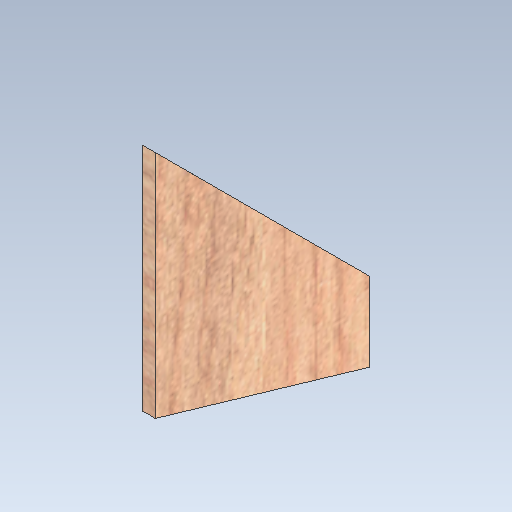
# Autodesk Inventor part: Aletas
Saved by Autodesk Inventor 2020 (Build 240168000, 168)
## iProperties
Created: 2021-10-16
Part Number: Aletas
Material: Birch
Document SubType Name: Modeling
Designer: Carlos
Density: 0.512 g/cm^3
Appearance: Birch - Natural Medium Gloss
Mass: 12.3724 g
Surface Area: 112.725 cm^2
Volume: 24.1649 cm^3
Author: Carlos
Autodesk Inventor part; units mm, degrees
ref_plane "YZ Plane" through (0, 0, 0) normal (1, 0, 0) x (0, 1, 0)
ref_plane "XZ Plane" through (0, 0, 0) normal (0, 1, 0) x (-1, 0, 0)
ref_plane "XY Plane" through (0, 0, 0) normal (0, 0, 1) x (1, 0, 0)
sketch "Sketch1" plane through (0, 0, 0) normal (1, 0, 0) x (0, 1, 0)
  line L0 (0, 0) -> (88, 0)
  line L1 (88, 0) -> (204.3575, 0) construction
  line L2 (88, 0) -> (6, -82)
  line L3 (88, 0) -> (171.4386, 0) construction
  line L4 (6, -82) -> (-24, -82)
  line L5 (-24, -82) -> (0, 0)
  dimension "d0" = 88
  dimension "d3" = 135
  dimension "d4" = 30
  constraints: 12 end point, 3 horizontal
  measures "d0" distance of L0.start L0.end
  measures "d3" angle of L2 L3
  measures "d4" distance of L2.end L4.end
extrude "Extrusion1" add sketch "Sketch1" against normal blind 5
sketch "Sketch2" plane through (0, 0, 0) normal (0, 1, 0) x (-1, 0, 0)
  line L0 (0, 0) -> (5, 0) projected
  circle A0 centre (2.5, 0) radius 36.5
  line L1 (0, 0) -> (0, -82) projected
  circle A1 centre (2.5, 36.5) radius 36.5855
  line L2 (5, -82) -> (5, 0) projected
  line L3 (0, 0) -> (5, 0)
  dimension "d7" = 73
  constraints: 2 end point, 1 horizontal, 1 midpoint, 1 vertical alignment, 5 other
extrude "Extrusion2" cut sketch "Sketch2" along normal mid plane 197.25 contours L0 A1
body "Solid1"
